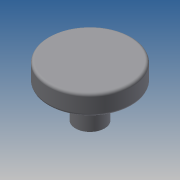
# Autodesk Inventor part: chimney
Saved by Autodesk Inventor 2014 SP1 (Build 180222100, 222)
## iProperties
Created: 2014-05-23
Part Number: chimney
Material: Generic
Document SubType Name: Modeling
Designer: Dave
Density: 1 g/cm^3
Appearance: Default
Author: Dave
Autodesk Inventor part; units mm, degrees
ref_plane "YZ Plane" through (0, 0, 0) normal (1, 0, 0) x (0, 1, 0)
sketch "Sketch1" plane through (0, 0, 0) normal (0, 1, 0) x (-1, 0, 0)
  circle A0 centre (0, 0) radius 76.2
  circle A1 centre (0, 0) radius 74.93
  dimension "d0" = 152.4
  dimension "d1" = 1.27
  constraints: 2 centre point, 1 coincident
  measures "d0" diameter of A0
  measures "d1" radial gap between concentric circles of A1 A0
extrude "Extrusion1" add sketch "Sketch1" along normal blind 203.2
sketch "Sketch2" plane through (0, 203.2, 0) normal (0, 1, 0) x (1, 0, 0)
  circle A0 centre (0, 0) radius 74.93 projected
  circle A1 centre (0, 0) radius 76.2 projected
  point P0 (0, 76.2)
  constraints: 1 vertical alignment, 1 other
ref_plane "Work Plane1" through (0, 203.2, -76.2) normal (0, 0, -1) x (-1, 0, 0)
sketch "Sketch3" plane through (0, 203.2, -76.2) normal (0, 0, -1) x (-1, 0, 0)
  line L0 (-6.3336, -31.75) -> (6.3664, -31.75)
  line L1 (6.3664, -31.75) -> (6.3664, -12.7)
  line L2 (6.3664, -12.7) -> (-6.3336, -12.7)
  line L3 (-6.3336, -12.7) -> (-6.3336, -31.75)
  line L4 (76.2, 0) -> (-76.2, 0) projected
  point P0 (0, -203.2)
  point P1 (0.0164, -12.7)
  dimension "d4" = 12.7
  dimension "d5" = 19.05
  dimension "d6" = 12.7
  constraints: 8 end point, 2 parallel, 1 horizontal, 1 midpoint, 1 perpendicular
  measures "d4" distance of L0.start L0.end
  measures "d5" distance of L2.end L0.start
  measures "d6" distance between parallel lines of L2 L4
extrude "Extrusion2" add sketch "Sketch3" along normal blind 1.27
sketch "Sketch4" plane through (0, 203.2, -77.47) normal (0, 0, -1) x (-1, 0, 0)
  line L0 (-6.3336, -31.75) -> (6.3664, -31.75) projected
  line L1 (6.3664, -31.75) -> (6.3664, -12.7) projected
  line L2 (-6.3336, -31.75) -> (6.3664, -31.75)
  line L3 (6.3664, -31.75) -> (6.3664, -30.48)
  line L4 (6.3664, -30.48) -> (-6.3336, -30.48)
  line L5 (-6.3336, -30.48) -> (-6.3336, -31.75)
  point P0 (0, -203.2)
  dimension "d9" = 1.27
  constraints: 8 end point, 2 parallel, 1 horizontal, 1 perpendicular, 1 point on line
  measures "d9" distance between parallel lines of L2 L4
extrude "Extrusion3" add sketch "Sketch4" along normal blind 101.6
pattern_circular "Circular Pattern1" count 3 over 360 about axis through (0, -10, 0) along (0, 1, 0) of "Extrusion2", "Extrusion3"
ref_plane "Work Plane5" through (-0.0164, 171.45, -76.2) normal (1, 0, 0) x (0, 0, -1)
sketch "Sketch8" plane through (-0.0164, 171.45, -76.2) normal (1, 0, 0) x (0, 0, -1)
  line L0 (91.2472, -0.0676) -> (129.3472, -0.0676)
  line L1 (142.0472, 12.6324) -> (142.0472, 88.8324)
  line L2 (129.3472, 101.5324) -> (-76.2, 101.5324)
  arc A0 (142.0472, 88.8324) -> (129.3472, 101.5324) centre (129.3472, 88.8324) ccw
  arc A1 (129.3472, -0.0676) -> (142.0472, 12.6324) centre (129.3472, 12.6324) ccw
  line L3 (-76.2, 102.8024) -> (129.3472, 102.8024)
  arc A2 (143.3172, 88.8324) -> (129.3472, 102.8024) centre (129.3472, 88.8324) ccw
  line L4 (143.3172, 88.8324) -> (143.3172, 12.6324)
  arc A3 (129.3472, -1.3376) -> (143.3172, 12.6324) centre (129.3472, 12.6324) ccw
  line L5 (129.3472, -1.3376) -> (91.2472, -1.3376)
  line L6 (-76.2, 101.5324) -> (-76.2, -188.2709) construction
  line L7 (91.2472, -1.3376) -> (91.2472, -0.0676)
  line L8 (-76.2, 101.5324) -> (-76.2, 102.8024)
  point P0 (-76.2, -171.45)
  point P1 (142.0472, -0.0676)
  point P2 (142.0472, 101.5324)
  dimension "d26" = 50.8
  dimension "d27" = 101.6
  dimension "d28" = 12.7
  dimension "d29" = 1.27
  constraints: 18 end point, 8 point on circle, 4 centre point, 4 parallel, 4 point on line, 4 tangent, 3 perpendicular, 1 equal radius, 1 horizontal, 4 other
  measures "d26" distance of L0.start point (142.047, -0.068)
  measures "d27" distance of point (142.047, -0.068) point (142.047, 101.532)
  measures "d28" radius of A0
  measures "d29" distance between parallel lines of L2 L3
revolve "Revolution3" add sketch "Sketch8" angle 360 about axis through (-0.0164, 272.9824, 0) along (0, -1, 0)
sketch "Sketch10" plane through (0, 203.2, 0) normal (0, 1, 0) x (1, 0, 0)
  circle A0 centre (0, 0) radius 82.55
  dimension "d34" = 165.1
  constraints: 1 centre point
  measures "d34" diameter of A0
extrude "Extrusion5" add sketch "Sketch10" along normal blind 6.35
sketch "Sketch11" plane through (0, 203.2, 0) normal (0, -1, 0) x (1, 0, 0)
  circle A0 centre (0, 0) radius 82.55 projected
  circle A1 centre (0, 0) radius 76.2 projected
extrude "Extrusion6" add sketch "Sketch11" along normal blind 12.7
body "Solid1"
